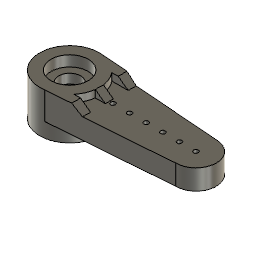
sg90 servo horn (Autodesk Fusion 360 design; units mm, degrees)
description: Spur Gear; Module: 1.0; Num Teeth: 36; Pressure Angle: 20.0; Backlash: 0.00 mm
Autodesk Fusion 360 part; units mm, degrees
sketch "Sketch4" plane through (0, 0, 0) normal (0, 0, 1) x (-1, 0, 0)
  circle A0 centre (-15.6, 0) radius 2.5
  line L0 (3.7, 0) -> (-18.1, 0) construction
  circle A1 centre (0, 0) radius 3.7
  line L1 (0, 0) -> (0, -3.7) construction
  line L2 (0, 0) -> (0, 3.7) construction
  line L3 (-15.6, 0) -> (-15.6, -2.5) construction
  line L4 (-15.6, 0) -> (-15.6, 2.5) construction
  line L5 (-15.6, -2.5) -> (0, -3.7)
  line L6 (-15.6, 2.5) -> (0, 3.7)
  circle A2 centre (0, 0) radius 1.35
  circle A3 centre (0, 0) radius 2.3
  circle A4 centre (-15.6, 0) radius 0.2875
  circle A5 centre (-13.55, 0) radius 0.2875
  circle A6 centre (-11.5, 0) radius 0.2875
  circle A7 centre (-9.45, 0) radius 0.2875
  circle A8 centre (-7.4, 0) radius 0.2875
  circle A9 centre (-5.35, 0) radius 0.2875
  point P0 (-15.6, 0)
  point P1 (-4.9, 0)
  dimension "d12" = 5
  dimension "d13" = 21.8
  dimension "d14" = 3.7
  dimension "d15" = 2.5
  dimension "d16" = 7.4
  dimension "d17" = 2.7
  dimension "d18" = 4.6
  dimension "d24" = 13.2
  dimension "d28" = 0.575
  dimension "d31" = -2.05
  dimension "d32" = 0
  constraint horizontal L0
  constraint coincident L0 A1.centre
  constraint coincident L0 P0
  constraint coincident P0 A0.centre
  constraint coincident A1.centre L1.start
  constraint coincident A1 L1.end
  constraint perpendicular L0 L1
  constraint coincident A1 L2.end
  constraint perpendicular L0 L2
  constraint coincident A0 L3.end
  constraint perpendicular L0 L3
  constraint coincident A0 L4.end
  constraint perpendicular L0 L4
  constraint concentric A1 A2
  constraint concentric A2 A3
  constraint coincident L0 P1
  measures "d12" diameter of A0
  measures "d13" distance of L0.start L0.end
  measures "d14" distance of L0.start A1.centre
  measures "d15" distance of L0.end P0
  measures "d16" diameter of A1
  measures "d17" diameter of A2
  measures "d18" diameter of A3
  measures "d24" distance of L0.end P1
  measures "d28" diameter of A4
extrude "Extrude3" add sketch "Sketch4" along normal blind 5.2 contours A1 L5 L6 | A1 L6 | A1 L5
extrude "Extrude4" add sketch "Sketch4" along normal blind 2.5 from surface at 1.8 contours A0 | A0 A1 L5 L6 | A4 | A5 | A6 | A7 | A8 | A9
extrude "Extrude5" add sketch "Sketch4" along normal blind 1.15 from surface at 2.75 contours A3
extrude "Extrude6" cut sketch "Sketch4" along normal through all contours A4 | A5 | A6 | A7 | A8 | A9
sketch "Sketch5" plane through (0, 0, 4.3) normal (0, 0, 1) x (-1, 0, 0)
  circle A0 centre (-9.45, 0) radius 0.2875
  circle A1 centre (-15.6, 0) radius 0.2875
  circle A2 centre (-7.4, 0) radius 0.2875
  circle A3 centre (-11.5, 0) radius 0.2875
  circle A4 centre (-13.55, 0) radius 0.2875
  circle A5 centre (-5.35, 0) radius 0.2875
  line L0 (-15.6, -2.5) -> (-0.5659, -3.6565)
  arc A6 (-0.5659, 3.6565) -> (-0.5659, -3.6565) centre (0, 0) ccw
  line L1 (-0.5659, 3.6565) -> (-15.6, 2.5)
  arc A7 (-15.6, 2.5) -> (-15.6, -2.5) centre (-15.6, 0) ccw
  line L2 (3.7, 0) -> (-18.1, 0)
  line L3 (-4.9, 0) -> (-4.9, -3.3231) construction
  line L4 (-4.9, 0) -> (-4.9, 3.3231) construction
  line L5 (-4.9, -2.3231) -> (2.8798, -2.3231)
  line L6 (-4.9, -0.5) -> (3.6661, -0.5)
  line L7 (-4.9, 0.5) -> (3.6661, 0.5)
  line L8 (-4.9, 2.3231) -> (2.8798, 2.3231)
  line L9 (-4.9, -3.3231) -> (-4.9, -2.3231)
  line L10 (-4.9, -0.5) -> (-4.9, 0.5)
  line L11 (-4.9, 2.3231) -> (-4.9, 3.3231)
  point P0 (-4.9, 0)
  dimension "d34" = 1
  dimension "d35" = 0.5
  dimension "d36" = 0.5
  dimension "d37" = 1
  constraint coincident P0 L3.start
  constraint coincident L0 L3.end
  constraint perpendicular L2 L3
  constraint coincident L1 L4.end
  constraint perpendicular L2 L4
  constraint coincident L3 L5.start
  constraint coincident A6 L5.end
  constraint perpendicular L3 L5
  constraint coincident L3 L6.start
  constraint coincident A6 L6.end
  constraint perpendicular L3 L6
  constraint coincident L4 L7.start
  constraint coincident A6 L7.end
  constraint perpendicular L4 L7
  constraint coincident L4 L8.start
  constraint coincident A6 L8.end
  constraint perpendicular L4 L8
  measures "d34" distance of L4.end L8
  measures "d35" distance of P0 L7
  measures "d36" distance of P0 L6
  measures "d37" distance of L3.end L5
extrude "Extrude7" add sketch "Sketch5" along normal up to surface (0.9 mm away) contours A6 L2 L7 L10 | A6 L2 L6 L10 | A6 L1 L8 L11 | L0 A6 L5 L9
ref_plane "WorkPlane1" through (4.283, -3.7, 4.75) normal (0, -1, 0) x (1, 0, 0)
sketch "Sketch7" plane through (0, -3.7, 0) normal (0, -1, 0) x (-1, 0, 0)
  line L0 (-4.9, -5.2) -> (-3.6661, -5.2)
  line L1 (-3.6661, -5.2) -> (-3.6661, -4.3)
  line L2 (-3.6661, -4.3) -> (-4.9, -4.3)
  line L3 (-4.9, -4.3) -> (-4.9, -5.2)
  line L4 (-3.6661, -5.2) -> (-4.9, -4.3)
  constraint coincident L0.end L1.start
  constraint coincident L2.end L3.start
extrude "Extrude8" cut sketch "Sketch7" against normal through all contours L0 L3 L4
equation "d14 = d16 / 2"
equation "d15 = d12 / 2"
equation "d36 = d35"
